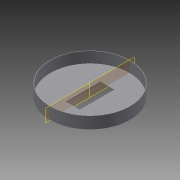
# Autodesk Inventor part: Top Cap
Saved by Autodesk Inventor 2015 (Build 190159000, 159)
## iProperties
Created: 2014-06-24
Part Number: Top Cap
Material: Generic
Document SubType Name: Modeling
Designer: Aki
Density: 1 g/cm^3
Appearance: Default
Author: Aki
Autodesk Inventor part; units mm, degrees
ref_plane "YZ Plane" through (0, 0, 0) normal (1, 0, 0) x (0, 1, 0)
ref_plane "XZ Plane" through (0, 0, 0) normal (0, 1, 0) x (-1, 0, 0)
ref_plane "XY Plane" through (0, 0, 0) normal (0, 0, 1) x (1, 0, 0)
sketch "Sketch1" plane through (0, 0, 0) normal (0, 1, 0) x (-1, 0, 0)
  circle A0 centre (0, 0) radius 87
  line L0 (-15, 37.5) -> (15, 37.5)
  line L1 (15, 37.5) -> (15, -37.5)
  line L2 (15, -37.5) -> (-15, -37.5)
  line L3 (-15, -37.5) -> (-15, 37.5)
  line L4 (-15, 37.5) -> (15, -37.5) construction
  line L5 (15, 37.5) -> (-15, -37.5) construction
  dimension "d1" = 174
  dimension "d41" = 30
  dimension "d42" = 75
  constraints: 12 end point, 2 midpoint, 2 parallel, 1 centre point, 1 horizontal, 1 perpendicular
  measures "d1" diameter of A0
  measures "d41" distance of L1.end L2.end
  measures "d42" distance of L0.end L1.end
extrude "Extrusion4" add sketch "Sketch1" along normal blind 25.4
sketch "Sketch4" plane through (0, 25.4, 0) normal (0, 1, 0) x (1, 0, 0)
  circle A0 centre (0, 0) radius 86
  dimension "d45" = 172
  constraints: 1 centre point, 1 coincident
  measures "d45" diameter of A0
hole "Hole2" at (0, 25.4, 0) direction (0, -1, 0) diameter 172 depth 23.4
ref_plane "Work Plane1" through (0, 0, 37.5) normal (1, 0, 0) x (0, 0, -1)
body "Solid3"
